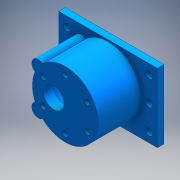
# Autodesk Inventor part: motorHolder57mmVer2
Saved by Autodesk Inventor 2016 (Build 200138000, 138)
## iProperties
Created: 2016-05-14
Part Number: motorHolder57mmVer2
Material: ABS Plastic
Document SubType Name: Modeling
Designer: hesaon
Density: 1.06 g/cm^3
Appearance: Smooth - White
Author: hesaon
Autodesk Inventor part; units mm, degrees
ref_plane "YZ Plane" through (0, 0, 0) normal (1, 0, 0) x (0, 1, 0)
ref_plane "XZ Plane" through (0, 0, 0) normal (0, 1, 0) x (-1, 0, 0)
ref_plane "XY Plane" through (0, 0, 0) normal (0, 0, 1) x (1, 0, 0)
sketch "Sketch1" plane through (0, 0, 0) normal (0, 1, 0) x (-1, 0, 0)
  circle A0 centre (0, 0) radius 19.95
  dimension "d0" = 39.9
  constraints: 1 centre point, 1 coincident
  measures "d0" diameter of A0
extrude "Extrusion1" add sketch "Sketch1" along normal blind 6
sketch "Sketch2" plane through (0, 6, 0) normal (0, 1, 0) x (1, 0, 0)
  circle A0 centre (0, 0) radius 19.95
  circle A1 centre (0, 0) radius 18.75
  dimension "d3" = 37.5
  dimension "d4" = 39.9
  constraints: 2 centre point, 2 coincident
  measures "d3" diameter of A1
  measures "d4" diameter of A0
extrude "Extrusion2" add sketch "Sketch2" along normal blind 20
sketch "Sketch3" plane through (0, 0, 0) normal (0, -1, 0) x (1, 0, 0)
  circle A0 centre (-7, 0) radius 6.25
  circle A1 centre (0, -15.5) radius 1.6
  circle A2 centre (13.4234, -7.75) radius 1.6
  circle A3 centre (13.4234, 7.75) radius 1.6
  circle A4 centre (0, 15.5) radius 1.6
  circle A5 centre (-13.4234, 7.75) radius 1.6
  circle A6 centre (-13.4234, -7.75) radius 1.6
  point P0 (0, 0)
  dimension "d7" = 0
  dimension "d8" = 7
  dimension "d9" = 12.5
  dimension "d10" = 3.2
  dimension "d11" = 0
  dimension "d12" = 15.5
  dimension "d15" = 360
  constraints: 7 centre point, 1 coincident, 13 other
  measures "d7" vertical distance of point (-7, 0) point (0, 0)
  measures "d8" distance of point (-7, 0) point (0, 0)
  measures "d9" diameter of A0
  measures "d10" diameter of A1
  measures "d11" horizontal distance of point (0, 0) A1.centre
  measures "d12" distance of point (0, 0) A1.centre
extrude "Extrusion3" cut sketch "Sketch3" against normal up to next
sketch "Sketch4" plane through (0, 26, 0) normal (0, 1, 0) x (1, 0, 0)
  circle A0 centre (0, 0) radius 18.75 projected
  line L0 (-29.9, -20.9) -> (29.9, -20.9)
  line L1 (29.9, -20.9) -> (29.9, 20.9)
  line L2 (29.9, 20.9) -> (-29.9, 20.9)
  line L3 (-29.9, 20.9) -> (-29.9, -20.9)
  line L4 (-29.9, -20.9) -> (29.9, 20.9) construction
  line L5 (29.9, -20.9) -> (-29.9, 20.9) construction
  dimension "d19" = 59.8
  dimension "d20" = 41.8
  constraints: 12 end point, 2 midpoint, 2 parallel, 1 horizontal, 1 perpendicular
  measures "d19" distance of L2.end L1.end
  measures "d20" distance of L1.end L0.end
extrude "Extrusion4" add sketch "Sketch4" along normal blind 4
sketch "Sketch5" plane through (0, 30, 0) normal (0, 1, 0) x (1, 0, 0)
  line L0 (29.9, -20.9) -> (29.9, 20.9) projected
  line L1 (-29.9, 20.9) -> (-29.9, -20.9) projected
  circle A0 centre (25, 15) radius 2.1
  circle A1 centre (25, 0) radius 2.1
  circle A2 centre (25, -15) radius 2.1
  circle A3 centre (-25, 15) radius 2.1
  circle A4 centre (-25, 0) radius 2.1
  circle A5 centre (-25, -15) radius 2.1
  point P0 (0, 0)
  dimension "d23" = 0
  dimension "d24" = 25
  dimension "d25" = 15
  dimension "d26" = 25
  dimension "d27" = 25
  dimension "d28" = 15
  dimension "d29" = 4.2
  dimension "d30" = 4.2
  dimension "d31" = 4.2
  dimension "d33" = 0
  dimension "d34" = 15
  dimension "d35" = 15
  dimension "d36" = 25
  dimension "d37" = 25
  dimension "d38" = 25
  dimension "d39" = 4.2
  dimension "d40" = 4.2
  dimension "d41" = 4.2
  constraints: 6 centre point, 6 coincident
  measures "d23" vertical distance of point (0, 0) point (25, 0)
  measures "d24" horizontal distance of point (25, -15) point (0, 0)
  measures "d25" vertical distance of point (0, 0) point (25, -15)
  measures "d26" distance of point (0, 0) point (25, 0)
  measures "d27" horizontal distance of point (0, 0) point (25, 15)
  measures "d28" distance of point (25, 0) point (25, 15)
  measures "d29" diameter of A0
  measures "d30" diameter of A1
  measures "d31" diameter of A2
  measures "d33" vertical distance of point (0, 0) point (-25, 0)
  measures "d34" distance of point (-25, 0) point (-25, -15)
  measures "d35" distance of point (-25, 0) point (-25, 15)
  measures "d36" horizontal distance of point (0, 0) point (-25, -15)
  measures "d37" distance of point (0, 0) point (-25, 0)
  measures "d38" horizontal distance of point (0, 0) point (-25, 15)
  measures "d39" diameter of A3
  measures "d40" diameter of A4
  measures "d41" diameter of A5
extrude "Extrusion5" cut sketch "Sketch5" against normal up to next
sketch "Sketch7" plane through (0, 26, 0) normal (0, -1, 0) x (1, 0, 0)
  line L0 (29.9, -20.9) -> (-29.9, -20.9) projected
  line L1 (14.3023, -9.9973) -> (16.3514, -11.4296)
  line L2 (-29.9, 20.9) -> (29.9, 20.9) projected
  line L3 (14.3023, 9.9973) -> (16.3514, 11.4296)
  circle A0 centre (0, 0) radius 19.95 projected
  arc A1 (18.3028, 7.9379) -> (13.7426, 14.4618) centre (16.3514, 11.4296) ccw
  arc A2 (13.7426, -14.4618) -> (18.3028, -7.9379) centre (16.3514, -11.4296) ccw
  arc A3 (-13.7426, 14.4618) -> (-18.3028, 7.9379) centre (-16.3514, 11.4296) ccw
  arc A4 (-18.3028, -7.9379) -> (-13.7426, -14.4618) centre (-16.3514, -11.4296) ccw
  line L4 (-16.3514, 11.4296) -> (-14.3023, 9.9973)
  line L5 (-14.3023, -9.9973) -> (-16.3514, -11.4296)
  dimension "d48" = 8
  dimension "d49" = 8
  dimension "d50" = 8
  dimension "d51" = 8
  dimension "d52" = 32.7028
  dimension "d53" = 32.7028
  dimension "d54" = 22.8591
  constraints: 8 end point, 8 point on circle, 4 centre point, 1 collinear, 13 other
  measures "d48" diameter of A1
  measures "d49" diameter of A2
  measures "d50" diameter of A3
  measures "d51" diameter of A4
  measures "d52" horizontal distance of L3.end L5.end
  measures "d53" horizontal distance of L1.end L4.start
  measures "d54" distance of L1.end L3.end
extrude "Extrusion8" add sketch "Sketch7" along normal blind 26 contours A0 A3 | A4 A0
body "Solid1"
